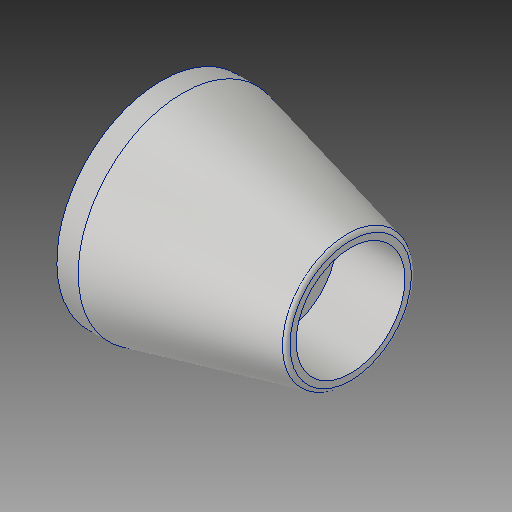
# Autodesk Inventor part: Pied
Saved by Autodesk Inventor 2017 (Build 210142000, 142)
## iProperties
Company: FABLAB Frenchmakers
Part Number: Pied
Material: Aluminium
Document SubType Name: Modeling
Designer: FABLAB Frenchmakers
Density: 2.7 g/cm^3
Appearance: Aluminium - Plat(2)
Mass: 15.9074 g
Surface Area: 26.1977 cm^2
Volume: 5.89162 cm^3
Stock Number: 1420-01-09
Project: 1420 Vauban 3D XL
Catalog Web Link: http://frenchmakers.com/
Autodesk Inventor part; units mm, degrees
ref_plane "YZ Plane" through (0, 0, 0) normal (1, 0, 0) x (0, 1, 0)
ref_plane "XZ Plane" through (0, 0, 0) normal (0, 1, 0) x (-1, 0, 0)
ref_plane "XY Plane" through (0, 0, 0) normal (0, 0, 1) x (1, 0, 0)
sketch "Esquisse1" plane through (0, 0, 0) normal (0, 0, 1) x (1, 0, 0)
  line L0 (-25.4342, 0) -> (0, 0)
  line L1 (-11.075, 3) -> (3.075, 3)
  line L2 (3.075, 3) -> (3.075, 6.375)
  line L3 (3.075, 6.375) -> (11.075, 6.375)
  line L4 (11.075, 6.375) -> (11.075, 7.1065)
  line L5 (10.6925, 7.5925) -> (-8.575, 12.25)
  line L6 (-8.575, 12.25) -> (-11.075, 12.25)
  line L7 (-11.075, 12.25) -> (-11.075, 3)
  arc A0 (11.075, 7.1065) -> (10.6925, 7.5925) centre (10.575, 7.1065) ccw
  point P0 (11.075, 7.5)
  dimension "d0" = 22.15
  dimension "d1" = 6
  dimension "d2" = 12.75
  dimension "d3" = 8
  dimension "d4" = 24.5
  dimension "d6" = 15
  dimension "d7" = 11.075
  dimension "d8" = 2.5
  dimension "d9" = 0.5
  constraints: 16 end point, 4 perpendicular, 2 horizontal, 2 point on circle, 2 point on line, 2 tangent, 1 centre point, 1 coincident, 1 parallel
  measures "d0" distance between parallel lines of L4 L7
  measures "d1" diameter of L1 L0
  measures "d2" diameter of L3 L0
  measures "d3" distance between parallel lines of L4 L2
  measures "d4" diameter of L6 L0
  measures "d6" diameter of point (11.075, 7.5) L0
  measures "d7" distance from line of point (0, 0) L7
  measures "d8" distance of L5.end L6.end
  measures "d9" radius of A0
revolve "Révolution1" add sketch "Esquisse1" angle 360 about axis through (-25.4342, 0, 0) along (1, 0, 0)
equation "\"d7\" = 0.5 * d0"
